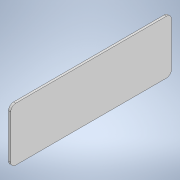
# Autodesk Inventor part: Conveyor Base
Saved by Autodesk Inventor 2022.2 (Build 262287000, 287)
## iProperties
Created: 2022-02-27
Part Number: Conveyor Base
Material: Generic
Document SubType Name: Modeling
Designer: PRASHANTH
Density: 1 g/cm^3
Appearance: Default
Author: PRASHANTH
Autodesk Inventor part; units mm, degrees
ref_plane "YZ Plane" through (0, 0, 0) normal (1, 0, 0) x (0, 1, 0)
ref_plane "XZ Plane" through (0, 0, 0) normal (0, 1, 0) x (-1, 0, 0)
ref_plane "XY Plane" through (0, 0, 0) normal (0, 0, 1) x (1, 0, 0)
sketch "Sketch1" plane through (0, 0, 0) normal (1, 0, 0) x (0, 1, 0)
  line L0 (-35.625, 180) -> (61.875, 180)
  line L1 (73.125, 168.75) -> (73.125, -168.75)
  line L2 (61.875, -180) -> (-35.625, -180)
  line L3 (-46.875, -168.75) -> (-46.875, 168.75)
  arc A0 (73.125, 168.75) -> (61.875, 180) centre (61.875, 168.75) ccw
  arc A1 (61.875, -180) -> (73.125, -168.75) centre (61.875, -168.75) ccw
  arc A2 (-46.875, -168.75) -> (-35.625, -180) centre (-35.625, -168.75) ccw
  arc A3 (-35.625, 180) -> (-46.875, 168.75) centre (-35.625, 168.75) ccw
  dimension "d5" = 360
  dimension "d6" = 120
  constraints: 8 end point, 8 point on circle, 8 tangent, 4 centre point, 3 equal radius, 2 parallel, 1 horizontal, 1 perpendicular
  measures "d5" distance between parallel lines of L2 L0
  measures "d6" distance between parallel lines of L3 L1
extrude "Extrusion1" add sketch "Sketch1" along normal blind 5
body "Solid1"
